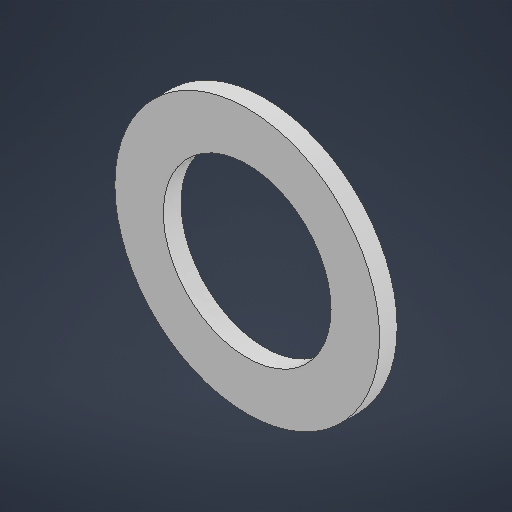
# Autodesk Inventor part: Spulenhalter-Abschluss-Ph-L
Saved by Autodesk Inventor 2026.1 (Build 301233000, 233)
## iProperties
Created: 2025-12-08
Part Number: Spulenhalter-Abschluss-Ph-L
Material: Generisch
Document SubType Name: Modeling
Designer: rebsa
Density: 1 g/cm^3
Appearance: Vorgabe
Author: rebsa
Autodesk Inventor part; units mm, degrees
ref_plane "YZ Plane" through (0, 0, 0) normal (1, 0, 0) x (0, 1, 0)
ref_plane "XZ Plane" through (0, 0, 0) normal (0, 1, 0) x (-1, 0, 0)
ref_plane "XY Plane" through (0, 0, 0) normal (0, 0, 1) x (1, 0, 0)
sketch "Skizze1" plane through (0, 0, 0) normal (0, 0, 1) x (1, 0, 0)
  line L0 (-21, 0) -> (21, 0) projected
  line L1 (0, -21) -> (0, 21) projected
  circle A0 centre (0, 0) radius 15
  circle A1 centre (0, 0) radius 9.5
  dimension "d0" = 19
  dimension "d1" = 30
  constraints: 2 centre point, 2 coincident
  measures "d0" diameter of A1
  measures "d1" diameter of A0
extrude "Extrusion1" add sketch "Skizze1" along normal blind 2 contours A1 L1 A0 L0 | L0 A0 L1 A1 | A1 L0 A0 L1 | L1 A0 L0 A1
